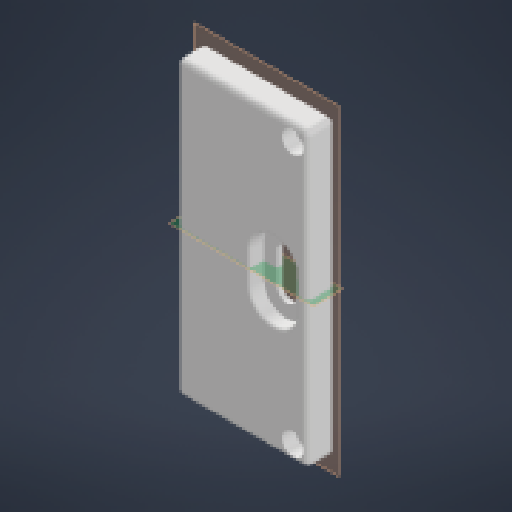
# Autodesk Inventor part: V2.0 Lid
Saved by Autodesk Inventor 2023 (Build 270158000, 158)
## iProperties
Created: 2022-12-23
Part Number: V2.0 Lid
Material: Generic
Document SubType Name: Modeling
Designer: User
Density: 1 g/cm^3
Appearance: Default
Author: User
Autodesk Inventor part; units mm, degrees
ref_plane "YZ Plane" through (0, 0, 0) normal (1, 0, 0) x (0, 1, 0)
ref_plane "XZ Plane" through (0, 0, 0) normal (0, 1, 0) x (-1, 0, 0)
ref_plane "Work Plane1" through (0, 0, 0) normal (0, 0, 1) x (1, 0, 0)
sketch "Sketch1" plane through (0, 0, 0) normal (0, 0, 1) x (1, 0, 0)
  circle A0 centre (9.2625, -24.1) radius 1.6 projected
  circle A1 centre (9.2625, 24.1) radius 1.6 projected
  line L0 (-12.0625, 26.9) -> (12.0625, 26.9) projected
  line L1 (-12.0625, 22.65) -> (-12.0625, 26.9) projected
  line L2 (-10.5625, 21.9) -> (-11.3125, 21.9) projected
  line L3 (-10.5625, 24.4) -> (-10.5625, 21.9) projected
  line L4 (-7.2375, 24.4) -> (-10.5625, 24.4) projected
  line L5 (-7.2375, 22.4) -> (-7.2375, 24.4) projected
  line L6 (2.0125, 22.4) -> (-7.2375, 22.4) projected
  line L7 (2.0125, 23.4) -> (2.0125, 22.4) projected
  line L8 (4.0625, 23.4) -> (2.0125, 23.4) projected
  line L9 (4.0625, 22.4) -> (4.0625, 23.4) projected
  line L10 (7.0376, 22.4) -> (4.0625, 22.4) projected
  arc A2 (7.0376, 22.4) -> (10.0625, 21.4167) centre (9.2625, 24.1) ccw projected
  line L11 (10.0625, -21.4167) -> (10.0625, 21.4167) projected
  arc A3 (10.0625, -21.4167) -> (7.0376, -22.4) centre (9.2625, -24.1) ccw projected
  line L12 (4.0625, -22.4) -> (7.0376, -22.4) projected
  line L13 (4.0625, -23.4) -> (4.0625, -22.4) projected
  line L14 (2.0125, -23.4) -> (4.0625, -23.4) projected
  line L15 (2.0125, -22.4) -> (2.0125, -23.4) projected
  line L16 (-7.2375, -22.4) -> (2.0125, -22.4) projected
  line L17 (-7.2375, -24.4) -> (-7.2375, -22.4) projected
  line L18 (-10.5625, -24.4) -> (-7.2375, -24.4) projected
  line L19 (-10.5625, -21.9) -> (-10.5625, -24.4) projected
  line L20 (-11.3125, -21.9) -> (-10.5625, -21.9) projected
  line L21 (-12.0625, -26.9) -> (-12.0625, -22.65) projected
  line L22 (12.0625, -26.9) -> (-12.0625, -26.9) projected
  line L23 (12.0625, 26.9) -> (12.0625, -26.9) projected
  line L24 (-12.0625, 21.9) -> (-10.5625, 21.9)
  line L25 (-10.5625, 21.9) -> (-10.5625, -21.9)
  line L26 (-10.5625, -21.9) -> (-12.0625, -21.9)
  line L27 (-12.0625, -21.9) -> (-12.0625, 21.9)
  line L28 (-7.2375, -22.4) -> (2.0125, -22.4)
  line L29 (2.0125, -22.4) -> (2.0125, 22.4)
  line L30 (2.0125, 22.4) -> (-7.2375, 22.4)
  line L31 (-7.2375, 22.4) -> (-7.2375, -22.4)
  line L32 (4.0625, 22.4) -> (10.0625, 22.4)
  line L33 (10.0625, 22.4) -> (10.0625, -22.4)
  line L34 (10.0625, -22.4) -> (4.0625, -22.4)
  line L35 (4.0625, -22.4) -> (4.0625, 22.4)
  line L36 (-12.0625, -22.65) -> (-11.3125, -21.9) projected
  line L37 (-11.3125, 21.9) -> (-12.0625, 22.65) projected
  line L38 (-12.0625, -26.9) -> (-12.0625, 26.9) projected
  point P0 (0, 0)
  point P1 (-12.0625, -21.9)
  constraints: 24 end point, 6 parallel, 3 horizontal, 3 perpendicular, 2 point on line
extrude "Extrusion1" add sketch "Sketch1" along normal blind 4.5 contours A0 | A1 | L0 L23 L22 L21 L36 L20 L19 L18 L17 L16 L15 L14 L13 L12 L34 L33 L11 L32 L10 L9 L8 L7 L6 L5 L4 L3 L2 L37 L1 | L37 L24 L38 | L2 L25 L20 L26 L27 L24 | L26 L36 L38 | L6 L29 L16 L31 | L10 A2 L11 A3 L12 L35 | L32 L33 A2 | A3 L33 L34
sketch "Sketch2" plane through (0, 0, 4.5) normal (0, 0, 1) x (1, 0, 0)
  line L0 (-12.0625, -26.9) -> (12.0625, -26.9) projected
  line L1 (12.0625, -26.9) -> (12.0625, 26.9) projected
  line L2 (12.0625, 26.9) -> (-12.0625, 26.9) projected
  line L3 (-10.5625, -24.4) -> (-10.5625, 24.4) projected
  line L4 (-10.5625, 24.4) -> (-7.2375, 24.4) projected
  line L5 (-7.2375, 24.4) -> (-7.2375, -24.4) projected
  line L6 (-7.2375, -24.4) -> (-10.5625, -24.4) projected
  line L7 (2.0125, -23.4) -> (2.0125, 23.4) projected
  line L8 (2.0125, 23.4) -> (4.0625, 23.4) projected
  line L9 (4.0625, 23.4) -> (4.0625, -23.4) projected
  line L10 (4.0625, -23.4) -> (2.0125, -23.4) projected
  line L11 (-12.0625, 26.9) -> (-12.0625, -26.9) projected
  point P0 (0, 0)
extrude "Extrusion2" add sketch "Sketch2" against normal blind 3.5 contours L7 L8 L9 L10
sketch "Sketch3" plane through (0, 0, 4.5) normal (0, 0, 1) x (1, 0, 0)
  line L0 (-7.2375, 24.4) -> (-7.2375, -24.4) projected
  line L1 (-10.5625, 24.4) -> (-7.2375, 24.4) projected
  line L2 (-10.5625, -24.4) -> (-10.5625, 24.4) projected
  line L3 (-7.2375, -24.4) -> (-10.5625, -24.4) projected
  point P0 (0, 0)
extrude "Extrusion3" add sketch "Sketch3" against normal blind 2.5
sketch "Sketch4" plane through (0, 0, 4.5) normal (0, 0, 1) x (1, 0, 0)
  circle A0 centre (9.2625, 24.1) radius 1.6 projected
  circle A1 centre (9.2625, -24.1) radius 1.6 projected
  circle A2 centre (9.2625, 24.1) radius 1.1
  circle A3 centre (9.2625, -24.1) radius 1.1
  point P0 (0, 0)
  dimension "d6" = 2.2
  dimension "d7" = 2.2
  constraints: 2 centre point, 2 coincident
  measures "d6" diameter of A2
  measures "d7" diameter of A3
extrude "Extrusion4" cut sketch "Sketch4" against normal up to next contours A2 | A3
sketch "Sketch5" plane through (0, 0, 4.5) normal (0, 0, 1) x (1, 0, 0)
  circle A0 centre (9.2625, 24.1) radius 1.1 projected
  circle A1 centre (9.2625, 24.1) radius 2
  circle A2 centre (9.2625, -24.1) radius 1.1 projected
  circle A3 centre (9.2625, -24.1) radius 2
  point P0 (0, 0)
  dimension "d10" = 4
  dimension "d11" = 4
  constraints: 2 centre point, 2 coincident
  measures "d10" diameter of A1
  measures "d11" diameter of A3
extrude "Extrusion5" cut sketch "Sketch5" against normal blind 2.5 contours A0 | A1 | A2 | A3
sketch "Sketch6" plane through (0, 0, 4.5) normal (0, 0, 1) x (1, 0, 0)
  line L0 (2.0125, -23.4) -> (2.0125, 23.4) projected
  line L1 (4.0625, 23.4) -> (4.0625, -23.4) projected
  line L2 (2.0125, -23.4) -> (2.0125, 23.4) projected
  line L3 (2.0125, 23.4) -> (4.0625, 23.4) projected
  line L4 (4.0625, -23.4) -> (2.0125, -23.4) projected
  line L5 (4.0625, 23.4) -> (4.0625, -23.4) projected
  line L6 (4.0625, -23.4) -> (4.0625, 6.6)
  line L7 (2.0125, 23.4) -> (4.0625, 23.4) projected
  line L8 (4.0625, 23.4) -> (4.0625, -6.6)
  line L9 (4.0625, -6.6) -> (8.9267, -6.6)
  line L10 (8.9267, -6.6) -> (8.9267, 6.6)
  line L11 (8.9267, 6.6) -> (4.0625, 6.6)
  arc A0 (7.2625, 2.9) -> (4.0625, 2.9) centre (5.6625, 2.9) ccw
  arc A1 (4.0625, -2.9) -> (7.2625, -2.9) centre (5.6625, -2.9) ccw
  line L12 (4.0625, -2.9) -> (4.0625, 2.9)
  line L13 (7.2625, 2.9) -> (7.2625, -2.9)
  arc A2 (7.4625, 2.9) -> (3.8625, 2.9) centre (5.6625, 2.9) ccw
  line L14 (7.4625, 2.9) -> (7.4625, -2.9)
  arc A3 (3.8625, -2.9) -> (7.4625, -2.9) centre (5.6625, -2.9) ccw
  line L15 (3.8625, -2.9) -> (3.8625, 2.9)
  line L16 (5.6625, 4.5) -> (5.6625, -6.6) construction
  line L17 (5.6625, -4.5) -> (5.6625, 6.6) construction
  point P0 (0, 0)
  dimension "d14" = 46.8
  dimension "d15" = 30
  dimension "d16" = 30
  dimension "d17" = 3.2
  dimension "d18" = 9
  dimension "d19" = 0.2
  constraints: 22 end point, 10 point on circle, 7 point on line, 4 centre point, 4 perpendicular, 4 tangent, 2 collinear, 2 parallel, 3 other
  measures "d14" distance of L1.start L1.end
  measures "d15" distance of L1.end L6.end
  measures "d16" distance of L1.start L8.end
  measures "d17" distance between parallel lines of L12 L13
  measures "d18" distance of L17.start L16.start
  measures "d19" radial gap between concentric circles of A0 A2
extrude "Extrusion6" cut sketch "Sketch6" against normal up to next contours A3 L15 A2 L1 | L1 A1 L13 A0 A2 L14 A3 | L1 A0 L13 A1
sketch "Sketch7" plane through (0, 0, 4.5) normal (0, 0, 1) x (1, 0, 0)
  arc A0 (3.8625, -2.9) -> (7.4625, -2.9) centre (5.6625, -2.9) ccw projected
  line L0 (3.8625, -2.9) -> (3.8625, 2.9) projected
  arc A1 (7.4625, 2.9) -> (3.8625, 2.9) centre (5.6625, 2.9) ccw projected
  line L1 (7.4625, 2.9) -> (7.4625, -2.9) projected
  circle A2 centre (9.2625, -24.1) radius 2 projected
  circle A3 centre (9.2625, 24.1) radius 2 projected
  line L2 (-12.0625, -26.9) -> (12.0625, -26.9) projected
  line L3 (12.0625, -26.9) -> (12.0625, 26.9) projected
  line L4 (12.0625, 26.9) -> (-12.0625, 26.9) projected
  line L5 (1.4125, 2.9) -> (1.4125, -2.9)
  arc A4 (1.4125, -2.9) -> (9.9125, -2.9) centre (5.6625, -2.9) ccw
  line L6 (9.9125, -2.9) -> (9.9125, 2.9)
  arc A5 (9.9125, 2.9) -> (1.4125, 2.9) centre (5.6625, 2.9) ccw
  line L7 (-12.0625, 26.9) -> (-12.0625, -26.9) projected
  point P0 (0, 0)
  dimension "d22" = 8.5
  constraints: 4 end point, 4 point on circle, 2 centre point, 3 other
  measures "d22" distance between parallel lines of L6 L5
extrude "Extrusion7" cut sketch "Sketch7" against normal blind 2.5 contours A5 L6 A4 L5
sketch "Sketch8" plane through (0, 0, 0) normal (0, 0, -1) x (-1, 0, 0)
  arc A0 (-1.4125, 2.9) -> (-9.9125, 2.9) centre (-5.6625, 2.9) ccw projected
  line L0 (-9.9125, 2.9) -> (-9.9125, -2.9) projected
  arc A1 (-9.9125, -2.9) -> (-1.4125, -2.9) centre (-5.6625, -2.9) ccw projected
  line L1 (-1.4125, -2.9) -> (-1.4125, 2.9) projected
  point P0 (0, 0)
extrude "Extrusion8" cut sketch "Sketch8" against normal blind 1
sketch "Sketch9" plane through (0, 0, 0) normal (0, 0, -1) x (-1, 0, 0)
  line L0 (11.3125, 21.9) -> (10.5625, 21.9) projected
  line L1 (10.5625, -21.9) -> (11.3125, -21.9) projected
  line L2 (12.0625, -26.9) -> (12.0625, 26.9) projected
  line L3 (10.5625, -24.4) -> (10.5625, 24.4) projected
  line L4 (12.0625, 26.9) -> (12.0625, -26.9) projected
  line L5 (12.0625, -21.9) -> (10.5625, -21.9)
  line L6 (10.5625, -21.9) -> (10.5625, 21.9)
  line L7 (10.5625, 21.9) -> (12.0625, 21.9)
  line L8 (12.0625, 21.9) -> (12.0625, -21.9)
  point P0 (0, 0)
  constraints: 8 end point, 2 parallel, 1 horizontal, 1 perpendicular, 1 point on line, 1 other
extrude "Extrusion9" add sketch "Sketch9" along normal blind 0.5
sketch "Sketch10" plane through (-12.0625, 21.9, 0) normal (0, 1, 0) x (1, 0, 0)
  line L0 (0, 0) -> (0, 0.5) projected
  line L1 (0, 0.5) -> (0, -0.25)
  line L2 (0, -0.25) -> (0.75, 0.5)
  line L3 (1.5, 0.5) -> (0, 0.5) projected
  line L4 (0.75, 0.5) -> (0, 0.5)
  point P0 (12.0625, 0)
  dimension "d29" = 0.75
  constraints: 6 end point, 1 collinear, 1 midpoint
  measures "d29" distance of L0.end L1.end
extrude "Extrusion10" cut sketch "Sketch10" against normal up to surface (43.8 mm away)
sketch "Sketch11" plane through (-10.5625, 21.9, 0) normal (0, 1, 0) x (1, 0, 0)
  line L0 (-0.75, 122.5) -> (-0.75, 0) projected
  line L1 (-0.75, 0.5) -> (-1.25, 0) projected
  line L2 (0, 0) -> (-1.25, 0) projected
  line L3 (-0.75, 122.5) -> (-0.75, 0)
  point P0 (10.5625, 0)
  point P1 (-1.5, -0.25)
  constraints: 2 end point, 1 vertical, 3 other
ref_plane "Work Plane2" through (-11.6875, 22.275, -123.25) normal (-0.7071068, -0.7071068, 0) x (0, 0, 1)
extrude "Extrusion11" add sketch "Sketch11" against normal up to surface surface through (-11.6875, 22.275, -123.25) normal (-0.7071068, -0.7071068, 0)
sketch "Sketch12" plane through (-12.0625, 21.9, 0) normal (0, -1, 0) x (1, 0, 0)
  line L0 (0.25, 0) -> (0, 0) projected
  line L1 (0, 0.25) -> (0.25, 0) projected
  line L2 (0, 0) -> (0, 0.25) projected
  point P0 (12.0625, 0)
extrude "Extrusion12" cut sketch "Sketch12" against normal up to surface surface through (-11.5625, 22.15, -0.25) normal (-0.7071068, -0.7071068, 0)
ref_plane "Work Plane3" through (-12.0625, 0, 0) normal (0, -1, 0) x (1, 0, 0)
mirror "Mirror1" about plane through (-12.0625, 0, 0) normal (0, -1, 0) of "Extrusion12", "Extrusion11"
fillet "Fillet1" radius 1 10 edges at (-12.0625, 26.9, 2.25) (0, 26.9, 4.5) (-12.0625, 2.5, 4.5) (-12.0625, -22.275, 4.5) (-12.0625, -24.775, 4.5) (12.0625, 26.9, 2.25) (12.0625, 0, 4.5) (0, -26.9, 4.5) (12.0625, -26.9, 2.25) (-12.0625, -26.9, 2.25)
fillet "Fillet2" radius 0.5 4 edges at (1.4125, 0, 4.5) (5.6625, 7.15, 4.5) (9.9125, 0, 4.5) (5.6625, -7.15, 4.5)
equation "\"d16\" = d15"
body "Solid1"
